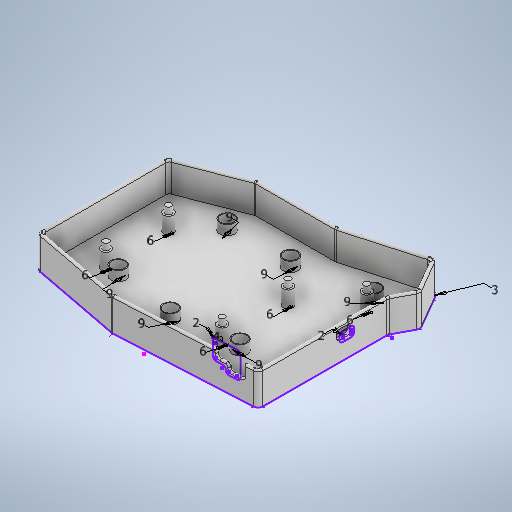
# Autodesk Inventor part: CASE_V1
Saved by Autodesk Inventor 2025 (Build 290162000, 162)
## iProperties
Created: 2025-01-14
Part Number: CASE_V1
Material: Типовые
Document SubType Name: Modeling
Designer: momop
Density: 1 g/cm^3
Appearance: По умолчанию
Author: momop
Autodesk Inventor part; units mm, degrees
ref_plane "YZ Plane" through (0, 0, 0) normal (1, 0, 0) x (0, 1, 0)
sketch "Эскиз1" plane through (0, 0, 0) normal (0, 1, 0) x (-1, 0, 0)
  circle A0 centre (-33.0003, 32.424) radius 4.0003
  circle A1 centre (-23.6143, 34.0744) radius 0.9002
  circle A2 centre (-23.6143, 34.0744) radius 1.8504
  circle A3 centre (4.9998, 37.4242) radius 3.9999
  circle A4 centre (43.9997, 30.4242) radius 3.9999
  circle A5 centre (52.3857, 29.5744) radius 0.8998
  circle A6 centre (52.3857, 29.5744) radius 1.8497
  circle A7 centre (-50.6142, -27.9253) radius 0.8999
  circle A8 centre (-50.6142, -27.9254) radius 1.85
  circle A9 centre (-47, -35.6735) radius 4
  circle A10 centre (-4.0003, -27.5756) radius 3.9999
  circle A11 centre (-23.6141, -6.4256) radius 0.9003
  circle A12 centre (-23.6144, -6.4251) radius 1.8498
  circle A13 centre (35, -27.5756) radius 3.9997
  circle A14 centre (52.3856, -8.9256) radius 1.8502
  circle A15 centre (52.3858, -8.9251) radius 0.8997
  line L0 (-60.6006, -55.9307) -> (-71.923, -36.2682)
  line L1 (-71.923, -36.2682) -> (-65.3386, -24.0646)
  line L2 (-65.3386, -24.0646) -> (-65.3386, 53.7044)
  line L3 (-65.3386, 53.7044) -> (16.6684, 59)
  line L4 (16.6684, 59) -> (71.8288, 47.4768)
  line L5 (71.8288, 47.4768) -> (71.8288, -28.4216)
  line L6 (71.8288, -28.4216) -> (33.8857, -42.9253)
  line L7 (33.8857, -42.9253) -> (-15.4601, -42.9253)
  line L8 (-15.4601, -42.9253) -> (-60.6006, -55.9307)
  circle A16 centre (52.3857, 29.5744) radius 3
  circle A17 centre (-23.6143, 34.0744) radius 3
  circle A18 centre (52.3856, -8.9256) radius 3
  circle A19 centre (-23.6141, -6.4256) radius 3
  circle A20 centre (-50.6142, -27.9254) radius 3
  circle A21 centre (-33.0003, 32.424) radius 4.5
  circle A22 centre (4.9998, 37.4242) radius 4.5
  circle A23 centre (43.9997, 30.4242) radius 4.5
  circle A24 centre (-47, -35.6735) radius 4.5
  circle A25 centre (-4.0003, -27.5756) radius 4.5
  circle A26 centre (35, -27.5756) radius 4.5
  point P0 (0, 0)
  dimension "d51" = 6
  dimension "d52" = 6
  dimension "d53" = 6
  dimension "d54" = 6
  dimension "d55" = 6
  dimension "d97" = 9
  dimension "d98" = 9
  dimension "d99" = 9
  dimension "d100" = 9
  dimension "d101" = 9
  dimension "d102" = 9
  constraints: 27 centre point, 18 end point, 12 coincident, 1 parallel, 1 perpendicular, 1 vertical
  measures "d51" diameter of A16
  measures "d52" diameter of A17
  measures "d53" diameter of A18
  measures "d54" diameter of A19
  measures "d55" diameter of A20
  measures "d97" diameter of A21
  measures "d98" diameter of A22
  measures "d99" diameter of A23
  measures "d100" diameter of A24
  measures "d101" diameter of A25
  measures "d102" diameter of A26
sketch "Эскиз2" plane through (0, 0, 0) normal (0, 1, 0) x (-1, 0, 0)
  line L0 (-51.0643, 55.2624) -> (-56.1361, 55.0644) projected
  ellipse E0 centre (-51.0642, 55.2625) end of major axis (-54.5661, 55.1259) minor radius 0.0002 projected
  ellipse E1 centre (-56.1362, 55.0645) end of major axis (-59.6383, 54.9278) minor radius 0.0001 projected
  ellipse E2 centre (-66.3395, 6.1174) end of major axis (-66.3395, 3.6172) minor radius 0 projected
  line L1 (-66.3395, 6.1175) -> (-66.3394, 2.0747) projected
  ellipse E3 centre (-66.3396, 2.0743) end of major axis (-66.3399, 4.574) minor radius 0.0001 projected
  point P0 (0, 0)
  constraints: 3 other
sketch "Эскиз3" plane through (0, 0, 0) normal (0, 1, 0) x (-1, 0, 0)
  line L0 (-72.4013, -35.2865) -> (-66.5401, -24.2557)
  line L1 (-66.3063, -23.3237) -> (-66.061, 52.4715)
  line L2 (-64.1669, 54.4622) -> (16.8665, 58.7561)
  line L3 (17.3505, 58.7228) -> (71.0167, 48.3894)
  line L4 (72.6386, 46.4259) -> (72.6532, -27.6161)
  line L5 (71.3747, -29.4818) -> (34.4308, -43.7711)
  line L6 (33.7098, -43.9058) -> (-14.625, -43.9154)
  line L7 (-15.9888, -44.1052) -> (-59.463, -56.4406)
  line L8 (-61.7383, -55.5212) -> (-72.3645, -37.2295)
  arc A0 (-64.1669, 54.4622) -> (-66.061, 52.4715) centre (-64.061, 52.465) ccw
  arc A1 (17.3505, 58.7228) -> (16.8665, 58.7561) centre (16.9723, 56.7589) ccw
  arc A2 (72.6386, 46.4259) -> (71.0167, 48.3894) centre (70.6386, 46.4255) ccw
  arc A3 (71.3747, -29.4818) -> (72.6532, -27.6161) centre (70.6532, -27.6165) ccw
  arc A4 (33.7098, -43.9058) -> (34.4308, -43.7711) centre (33.7094, -41.9058) ccw
  arc A5 (-61.7383, -55.5212) -> (-59.463, -56.4406) centre (-60.009, -54.5166) ccw
  arc A6 (-72.4013, -35.2865) -> (-72.3645, -37.2295) centre (-70.6352, -36.2249) ccw
  arc A7 (-66.5401, -24.2557) -> (-66.3063, -23.3237) centre (-68.3063, -23.3172) ccw
  arc A8 (-14.625, -43.9154) -> (-15.9888, -44.1052) centre (-14.624, -48.9154) ccw
  line L9 (-37.18, -52.197) -> (-15.4429, -46.0293)
  line L10 (9.5428, -45.9106) -> (-14.6246, -45.9154)
  line L11 (9.5428, -45.9106) -> (33.8967, -45.9058)
  line L12 (53.6243, -38.4918) -> (34.9783, -45.7038)
  line L13 (53.6243, -38.4918) -> (72.7356, -31.0998)
  line L14 (74.6459, 9.4053) -> (74.6533, -28.3012)
  line L15 (74.6459, 9.4053) -> (74.6384, 47.2519)
  line L16 (44.5617, 55.5201) -> (72.2056, 50.1972)
  line L17 (-23.756, 58.6064) -> (16.8827, 60.7598)
  line L18 (-23.756, 58.6064) -> (-65.2167, 56.4094)
  line L19 (-68.1836, 14.5804) -> (-68.058, 53.4233)
  line L20 (-71.2369, -28.8326) -> (-68.6546, -23.9728)
  line L21 (-71.2369, -28.8326) -> (-74.4283, -34.8389)
  line L22 (-68.7808, -47.38) -> (-74.3731, -37.7535)
  line L23 (-68.7808, -47.38) -> (-63.0774, -57.1976)
  line L24 (-37.18, -52.197) -> (-59.6645, -58.5767)
  line L25 (-68.1836, 14.5804) -> (-68.3039, -22.5749)
  line L26 (44.5617, 55.5201) -> (17.6086, 60.7099)
  arc A9 (-63.0774, -57.1976) -> (-59.6645, -58.5767) centre (-60.4834, -55.6907) ccw
  arc A10 (-74.4283, -34.8389) -> (-74.3731, -37.7535) centre (-71.7791, -36.2466) ccw
  arc A11 (-68.6546, -23.9728) -> (-68.3039, -22.5749) centre (-71.3038, -22.5651) ccw
  arc A12 (-65.2167, 56.4094) -> (-68.058, 53.4233) centre (-65.058, 53.4136) ccw
  arc A13 (17.6086, 60.7099) -> (16.8827, 60.7598) centre (17.0414, 57.764) ccw
  arc A14 (74.6384, 47.2519) -> (72.2056, 50.1972) centre (71.6384, 47.2514) ccw
  arc A15 (72.7356, -31.0998) -> (74.6533, -28.3012) centre (71.6533, -28.3018) ccw
  arc A16 (33.8967, -45.9058) -> (34.9783, -45.7038) centre (33.8961, -42.9058) ccw
  arc A17 (-14.6246, -45.9154) -> (-15.4429, -46.0293) centre (-14.624, -48.9154) ccw
  point P0 (0, 0)
  dimension "d96" = 3
  constraints: 54 end point, 36 point on circle, 34 tangent, 18 centre point, 14 equal radius, 13 parallel, 1 perpendicular
  measures "d96" radius of A9
extrude "Выдавливание3" add sketch "Эскиз1" along normal blind 12 contours A1 | A2 | A5 | A6 | A7 | A8 | A11 | A12 | A14 | A15 | A16 | A17 | A18 | A19 | A20
extrude "Выдавливание4" add sketch "Эскиз1" along normal blind 16 contours A1 | A2 | A5 | A6 | A7 | A8 | A11 | A12 | A14 | A15
ref_plane "РабПлоскость4" through (65.4819, 0, 58.7104) normal (0.0526875, 0, 0.998611) x (0.998611, 0, -0.0526875)
sketch "Эскиз6" plane through (65.4819, 0, 58.7104) normal (0.0526875, 0, 0.998611) x (0.998611, 0, -0.0526875)
  line L0 (-16.2159, 16) -> (-17.7203, 16)
  line L1 (-17.7203, 16) -> (-19.7203, 16)
  line L2 (-21.7203, 18) -> (-21.7203, 25.9822)
  line L3 (-19.7203, 27.9822) -> (-17.7203, 27.9822)
  line L4 (-17.7203, 27.9822) -> (-7.6362, 27.9822)
  line L5 (-5.6362, 25.9822) -> (-5.6362, 16)
  line L6 (-5.6362, 16) -> (-5.6362, 14)
  line L7 (-7.6362, 12) -> (-12.2159, 12)
  line L8 (-14.2159, 14) -> (-14.2159, 14)
  arc A0 (-19.7203, 27.9822) -> (-21.7203, 25.9822) centre (-19.7203, 25.9822) ccw
  arc A1 (-21.7203, 18) -> (-19.7203, 16) centre (-19.7203, 18) ccw
  arc A2 (-14.2159, 14) -> (-16.2159, 16) centre (-16.2159, 14) ccw
  arc A3 (-14.2159, 14) -> (-12.2159, 12) centre (-12.2159, 14) ccw
  arc A4 (-7.6362, 12) -> (-5.6362, 14) centre (-7.6362, 14) ccw
  arc A5 (-5.6362, 25.9822) -> (-7.6362, 27.9822) centre (-7.6362, 25.9822) ccw
  point P0 (-62.2976, 0)
  point P1 (-21.7203, 27.9822)
  point P2 (-14.2159, 14)
  dimension "d74" = 4
  dimension "d75" = 2
  constraints: 18 end point, 12 point on circle, 12 tangent, 6 centre point, 5 equal radius, 2 horizontal, 2 perpendicular, 2 point on line, 1 parallel
  measures "d74" distance of point (-21.72, 27.982) L3.end
  measures "d75" radius of A0
extrude "Выдавливание8" cut sketch "Эскиз6" against normal blind 24
ref_plane "РабПлоскость1" through (70.3386, 0, 56.6277) normal (1, 0, 0) x (0, 0, -1)
sketch "Эскиз7" plane through (70.3386, 0, 56.6277) normal (1, 0, 0) x (0, 0, -1)
  line L0 (50.5103, 12) -> (50.0101, 12)
  line L1 (48.0101, 15.2) -> (48.0101, 14.6)
  line L2 (50.5103, 17.8514) -> (55.0529, 17.8514)
  line L3 (57.0529, 14) -> (57.0529, 15.8514)
  arc A0 (57.0529, 15.8514) -> (55.0529, 17.8514) centre (55.0529, 15.8514) ccw
  arc A1 (55.0529, 12) -> (57.0529, 14) centre (55.0529, 14) ccw
  arc A2 (48.0101, 14) -> (50.0101, 12) centre (50.0101, 14) ccw
  line L4 (48.0101, 14) -> (48.0101, 14.6)
  line L5 (50.5103, 12) -> (55.0529, 12)
  line L6 (50.5103, 17.8514) -> (50.0101, 17.8514)
  line L7 (48.0101, 15.8514) -> (48.0101, 15.2)
  arc A3 (50.0101, 17.8514) -> (48.0101, 15.8514) centre (50.0101, 15.8514) ccw
  dimension "d86" = 2
  constraints: 16 end point, 8 point on circle, 6 tangent, 4 centre point, 3 horizontal, 1 equal radius, 1 perpendicular, 1 vertical
  measures "d86" radius of A3
extrude "Выдавливание9" cut sketch "Эскиз7" against normal blind 24
extrude "Выдавливание10" add sketch "Эскиз3" along normal blind 2 contours L0 A7 L1 A0 L2 A1 L3 A2 L4 A3 L5 A4 L6 A8 L7 A5 L8 A6 | L24 A9 L23 L22 A10 L21 L20 A11 L25 L19 A12 L18 L17 A13 L26 L16 A14 L15 L14 A15 L13 L12 A16 L11 L10 A17 L9
extrude "Выдавливание11" add sketch "Эскиз1" along normal blind 8 contours A21 | A22 | A23 | A24 | A25 | A26
extrude "Выдавливание12" cut sketch "Эскиз1" along normal blind 8 contours A0 | A3 | A4 | A9 | A10 | A13
extrude "Выдавливание13" add sketch "Эскиз3" along normal blind 20
extrude "Выдавливание14" cut sketch "Эскиз7" against normal blind 20
extrude "Выдавливание15" cut sketch "Эскиз6" against normal blind 20
fillet "Сопряжение5" radius 1 53 edges at (-17.1095, 20, 58.7542) (-44.1836, 20, 53.5561) (-72.1806, 20, 47.6992) (-72.6459, 20, 9.4049) (-72.303, 20, -28.747) (-52.9028, 20, -36.6265) (-34.0765, 20, -43.8718) (-9.5424, 20, -43.9106) (15.3134, 20, -43.9631) (37.7259, 20, -50.2729) (60.7583, 20, -56.3709) (67.0514, 20, -46.3754) (72.6348, 20, -36.2628) (69.4707, 20, -29.7711) (66.3664, 20, -23.8039) (66.1837, 20, 14.5739) (65.51, 20, 53.8437) (61.8967, 20, 54.5825) (13.3492, 20, 57.155) (-17.2472, 20, 60.7569) (-44.9071, 20, 55.4536) (-73.9514, 20, 49.1619) (-74.6459, 20, 9.4754) (-74.1281, 20, -29.9977) (-53.857, 20, -38.4018) (-34.4469, 20, -45.8548) (-9.6361, 20, -45.9106) (15.0377, 20, -45.944) (37.5537, 20, -52.303) (61.6074, 20, -58.4722) (68.7253, 20, -47.4756) (74.7785, 20, -36.3034) (71.5415, 20, -29.4059) (68.394, 20, -23.2952) (68.1809, 20, 15.4242) (67.2314, 20, 55.4815) (13.3938, 20, 59.1555) (50.4738, 15.4142, 55.1878) (51.6437, 12.5858, 55.1258) (55.3426, 12, 54.9298) (59.0415, 12.5858, 54.7338) (59.6265, 17, 54.7028) (44.1498, 16.5858, 55.5229) (43.5649, 19, 55.5539) (47.3118, 16, 55.3554) (44.2552, 16.5858, 57.5201) (43.6702, 19, 57.5511) (50.5792, 15.4142, 57.185) (51.7491, 12.5858, 57.123) (55.448, 12, 56.927) (59.1469, 12.5858, 56.731) (59.7318, 17, 56.7) (47.4172, 16, 57.3526)
